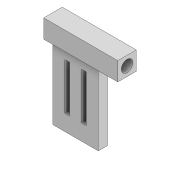
# Autodesk Inventor part: 20210811_H2_gasmanifold_old_v1
Saved by Autodesk Inventor 2022 (Build 260153000, 153)
## iProperties
Created: 2021-08-11
Part Number: 20210811_H2_gasmanifold_old_v1
Material: Generic
Document SubType Name: Modeling
Designer: scott
Density: 1 g/cm^3
Appearance: Default
Author: scott
Autodesk Inventor part; units mm, degrees
ref_plane "YZ Plane" through (0, 0, 0) normal (1, 0, 0) x (0, 1, 0)
ref_plane "XZ Plane" through (0, 0, 0) normal (0, 1, 0) x (-1, 0, 0)
ref_plane "XY Plane" through (0, 0, 0) normal (0, 0, 1) x (1, 0, 0)
sketch "Sketch1" plane through (0, 0, 0) normal (0, 1, 0) x (-1, 0, 0)
  line L0 (0, 0) -> (-19.6, 0)
  line L1 (-19.6, 0) -> (-19.6, -4)
  line L2 (-19.6, -4) -> (0, -4)
  line L3 (0, -4) -> (0, 0)
  dimension "d0" = 4
  dimension "d1" = 19.6
  constraints: 8 end point, 2 parallel, 1 horizontal, 1 perpendicular
  measures "d0" distance of L0.end L1.end
  measures "d1" distance of L1.end L2.end
extrude "Extrusion1" add sketch "Sketch1" along normal blind 34
sketch "Sketch2" plane through (0, 0, -4) normal (-1, 0, 0) x (0, 0, 1)
  line L0 (4, 34) -> (0, 34) projected
  line L1 (0, 34) -> (8, 34)
  line L2 (8, 34) -> (8, 42)
  line L3 (8, 42) -> (0, 42)
  line L4 (0, 42) -> (0, 34)
  line L5 (4, 0) -> (4, 34) projected
  dimension "d4" = 4
  dimension "d5" = 8
  dimension "d6" = 8
  constraints: 8 end point, 2 parallel, 1 horizontal, 1 perpendicular
  measures "d4" distance between parallel lines of L2 L5
  measures "d5" distance of L1.end L2.end
  measures "d6" distance of L2.end L3.end
extrude "Extrusion2" add sketch "Sketch2" against normal blind 32
sketch "Sketch3" plane through (32, 0, -4) normal (1, 0, 0) x (0, 0, -1)
  circle A0 centre (-4, 38) radius 2.5
  line L0 (0, 42) -> (-8, 42) projected
  line L1 (-8, 42) -> (-8, 34) projected
  line L2 (0, 34) -> (0, 42) projected
  line L3 (-8, 34) -> (0, 34) projected
  point P0 (-4, 0)
  dimension "d9" = 4
  dimension "d10" = 4
  dimension "d11" = 4
  dimension "d12" = 4
  dimension "d13" = 5
  constraints: 1 centre point
  measures "d9" distance from line of L0 A0.centre
  measures "d10" distance from line of L1 A0.centre
  measures "d11" distance from line of L2 A0.centre
  measures "d12" distance from line of L3 A0.centre
  measures "d13" diameter of A0
extrude "Extrusion3" cut sketch "Sketch3" against normal blind 30.8 contours A0
sketch "Sketch4" plane through (0, 0, 0) normal (0, -1, 0) x (1, 0, 0)
  line L0 (18.4, -3.2) -> (15.6, -3.2)
  line L1 (15.6, -3.2) -> (15.6, -1.6)
  line L2 (15.6, -1.6) -> (18.4, -1.6)
  line L3 (18.4, -1.6) -> (18.4, -3.2)
  line L4 (11.2, -3.2) -> (8.4, -3.2)
  line L5 (8.4, -3.2) -> (8.4, -1.6)
  line L6 (8.4, -1.6) -> (11.2, -1.6)
  line L7 (11.2, -1.6) -> (11.2, -3.2)
  line L8 (4, -3.2) -> (1.2, -3.2)
  line L9 (1.2, -3.2) -> (1.2, -1.6)
  line L10 (1.2, -1.6) -> (4, -1.6)
  line L11 (4, -1.6) -> (4, -3.2)
  line L12 (19.6, 0) -> (19.6, -4) projected
  line L13 (19.6, -4) -> (0, -4) projected
  line L14 (0, 0) -> (19.6, 0) projected
  line L15 (0, -4) -> (0, 0) projected
  dimension "d16" = 2.8
  dimension "d17" = 1.2
  dimension "d18" = 0.8
  dimension "d19" = 1.6
  dimension "d20" = 1.6
  dimension "d21" = 2.8
  dimension "d22" = 2.8
  dimension "d23" = 4.4
  dimension "d24" = 1.2
  dimension "d25" = 4.4
  constraints: 24 end point, 6 parallel, 4 point on line, 3 horizontal, 3 perpendicular
  measures "d16" distance of L1.end L2.end
  measures "d17" distance between parallel lines of L12 L3
  measures "d18" distance between parallel lines of L13 L0
  measures "d19" distance of L2.end L0.start
  measures "d20" distance between parallel lines of L14 L2
  measures "d21" distance of L5.end L6.end
  measures "d22" distance of L9.end L10.end
  measures "d23" distance between parallel lines of L7 L1
  measures "d24" distance between parallel lines of L15 L9
  measures "d25" distance between parallel lines of L11 L5
extrude "Extrusion4" cut sketch "Sketch4" against normal blind 38 contours L0 L1 L2 L3 | L4 L5 L6 L7 | L8 L9 L10 L11
sketch "Sketch5" plane through (19.6, 0, -4) normal (0, 0, -1) x (-1, 0, 0)
  line L0 (1.2, 0) -> (1.2, 38) projected
  line L1 (4, 0) -> (4, 38) projected
  line L2 (1.2, 27) -> (4, 27)
  line L3 (4, 27) -> (4, 7)
  line L4 (4, 7) -> (1.2, 7)
  line L5 (1.2, 7) -> (1.2, 27)
  line L6 (8.4, 0) -> (8.4, 36.0791) projected
  line L7 (11.2, 0) -> (11.2, 38) projected
  line L8 (8.4, 27) -> (11.2, 27)
  line L9 (11.2, 27) -> (11.2, 7)
  line L10 (11.2, 7) -> (8.4, 7)
  line L11 (8.4, 7) -> (8.4, 27)
  line L12 (15.6, 0) -> (15.6, 36.0791) projected
  line L13 (15.6, 27) -> (18.4, 27)
  line L14 (18.4, 27) -> (18.4, 7)
  line L15 (18.4, 7) -> (15.6, 7)
  line L16 (15.6, 7) -> (15.6, 27)
  line L17 (0, 0) -> (19.6, 0) projected
  line L18 (0, 34) -> (-12.4, 34) projected
  line L19 (19.6, 0) -> (19.6, 42) projected
  point P0 (18.4, 0)
  point P1 (15.6, 7)
  point P2 (8.4, 7)
  point P3 (1.2, 7)
  point P4 (4, 27)
  dimension "d28" = 7
  dimension "d29" = 20
  dimension "d30" = 7
  dimension "d49" = 1.2
  constraints: 24 end point, 9 point on line, 6 parallel, 3 horizontal, 3 perpendicular
  measures "d28" distance between parallel lines of L17 L4
  measures "d29" distance between parallel lines of L4 L2
  measures "d30" distance between parallel lines of L18 L2
  measures "d49" distance between parallel lines of L19 L14
extrude "Extrusion5" cut sketch "Sketch5" against normal blind 0.8 contours L12 L13 L14 L15 | L0 L2 L1 L4 | L6 L8 L7 L10
sketch "Sketch6" plane through (19.6, 0, -4) normal (0, 0, -1) x (-1, 0, 0)
  line L0 (5.2, 27) -> (7.2, 27)
  line L1 (7.2, 27) -> (7.2, 7)
  line L2 (7.2, 7) -> (5.2, 7)
  line L3 (5.2, 7) -> (5.2, 27)
  line L4 (12.4, 27) -> (14.4, 27)
  line L5 (14.4, 27) -> (14.4, 7)
  line L6 (14.4, 7) -> (12.4, 7)
  line L7 (12.4, 7) -> (12.4, 27)
  line L8 (4, 27) -> (4, 7) projected
  line L9 (8.4, 7) -> (8.4, 27) projected
  line L10 (11.2, 27) -> (11.2, 7) projected
  line L11 (15.6, 7) -> (15.6, 27) projected
  line L12 (19.6, 0) -> (19.6, 42) projected
  line L13 (0, 0) -> (0, 34) projected
  dimension "d33" = 1.2
  dimension "d34" = 1.2
  dimension "d35" = 1.2
  dimension "d36" = 1.2
  dimension "d37" = 2
  dimension "d38" = 2
  dimension "d39" = 19.6
  constraints: 16 end point, 4 parallel, 2 horizontal, 2 perpendicular, 2 point on line
  measures "d33" distance between parallel lines of L3 L8
  measures "d34" distance between parallel lines of L9 L1
  measures "d35" distance between parallel lines of L7 L10
  measures "d36" distance between parallel lines of L11 L5
  measures "d37" distance of L0.start L0.end
  measures "d38" distance of L4.start L4.end
  measures "d39" distance between parallel lines of L12 L13
extrude "Extrusion6" cut sketch "Sketch6" against normal up to surface (4 mm away)
sketch "Sketch7" plane through (0, 0, 0) normal (0, -1, 0) x (1, 0, 0)
  line L0 (19.6, -4) -> (32, -4) projected
  line L1 (0, 0) -> (19.6, 0) projected
  line L2 (19.6, -4) -> (0, -4)
  line L3 (0, -4) -> (0, 0)
  line L4 (0, 0) -> (19.6, 0)
  line L5 (19.6, 0) -> (19.6, -4)
  constraints: 8 end point, 2 parallel, 1 horizontal, 1 perpendicular
extrude "Extrusion7" add sketch "Sketch7" against normal blind 7
body "Solid1"
